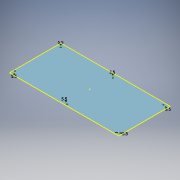
# Autodesk Inventor part: 240710_part3
Saved by Autodesk Inventor 2016 (Build 200138000, 138)
## iProperties
Created: 2024-07-10
Part Number: 240710_part3
Material: 일반
Document SubType Name: Modeling
Designer: pc
Density: 1 g/cm^3
Appearance: 기본값(1)
Author: pc
Autodesk Inventor part; units mm, degrees
ref_plane "YZ Plane" through (0, 0, 0) normal (1, 0, 0) x (0, 1, 0)
ref_plane "XZ Plane" through (0, 0, 0) normal (0, 1, 0) x (-1, 0, 0)
ref_plane "XY Plane" through (0, 0, 0) normal (0, 0, 1) x (1, 0, 0)
sketch "스케치1" plane through (0, 0, 0) normal (0, 0, 1) x (1, 0, 0)
  line L0 (250, -117.5) -> (-250, -117.5)
  line L1 (-250, -117.5) -> (-250, 117.5)
  line L2 (-250, 117.5) -> (250, 117.5)
  line L3 (250, 117.5) -> (250, -117.5)
  line L4 (250, -117.5) -> (-250, 117.5) construction
  line L5 (-250, -117.5) -> (250, 117.5) construction
  point P0 (0, 0)
  dimension "d0" = 500
  dimension "d1" = 235
  constraints: 12 end point, 2 midpoint, 2 parallel, 1 horizontal, 1 perpendicular
  measures "d0" distance of L1.end L2.end
  measures "d1" distance of L0.end L1.end
extrude "돌출1" add sketch "스케치1" along normal blind 1.2
sketch "스케치2" plane through (0, 0, 1.2) normal (0, 0, 1) x (1, 0, 0)
  line L0 (-250, -117.5) -> (250, -117.5) projected
  line L1 (250, -117.5) -> (250, 117.5) projected
  line L2 (250, 117.5) -> (-250, 117.5) projected
  line L3 (-250, 117.5) -> (-250, -117.5) projected
  point P0 (0, 0)
sketch "스케치3" plane through (0, 0, 1.2) normal (0, 0, 1) x (1, 0, 0)
  line L0 (-250, -117.5) -> (250, -117.5) projected
  line L1 (250, -117.5) -> (250, 117.5) projected
  line L2 (250, 117.5) -> (-250, 117.5) projected
  line L3 (-250, 117.5) -> (-250, -117.5) projected
  point P0 (0, 0)
sketch "스케치4" plane through (0, 0, 1.2) normal (0, 0, 1) x (1, 0, 0)
  line L0 (-250, -117.5) -> (250, -117.5) projected
  line L1 (250, -117.5) -> (250, 117.5) projected
  line L2 (250, 117.5) -> (-250, 117.5) projected
  line L3 (-250, 117.5) -> (-250, -117.5) projected
  point P0 (0, 0)
sketch "스케치5" plane through (0, 0, 1.2) normal (0, 0, 1) x (1, 0, 0)
  line L0 (-250, -117.5) -> (250, -117.5) projected
  line L1 (250, -117.5) -> (250, 117.5) projected
  line L2 (250, 117.5) -> (-250, 117.5) projected
  line L3 (-250, 117.5) -> (-250, -117.5) projected
  circle A0 centre (-238.0339, 105.4556) radius 2.75
  circle A1 centre (0, 105.4556) radius 2.75
  circle A2 centre (237.9578, 105.4556) radius 2.75
  circle A3 centre (237.9578, -105.56) radius 2.75
  circle A4 centre (0, -105.56) radius 2.75
  circle A5 centre (-238.0339, -105.56) radius 2.75
  point P0 (0, 0)
  dimension "d4" = 5.5
  dimension "d5" = 5.5
  dimension "d6" = 5.5
  dimension "d7" = 5.5
  dimension "d8" = 5.5
  dimension "d9" = 5.5
  constraints: 6 centre point
  measures "d4" diameter of A0
  measures "d5" diameter of A1
  measures "d6" diameter of A2
  measures "d7" diameter of A3
  measures "d8" diameter of A4
  measures "d9" diameter of A5
